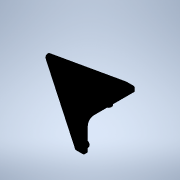
# Autodesk Inventor part: gato
Saved by Autodesk Inventor 2021 (Build 250183000, 183)
## iProperties
Created: 2024-10-06
Part Number: gato
Material: Generic
Document SubType Name: Modeling
Designer: hojan
Density: 1 g/cm^3
Appearance: Default
Author: hojan
Autodesk Inventor part; units mm, degrees
ref_plane "YZ Plane" through (0, 0, 0) normal (1, 0, 0) x (0, 1, 0)
ref_plane "XZ Plane" through (0, 0, 0) normal (0, 1, 0) x (-1, 0, 0)
ref_plane "XY Plane" through (0, 0, 0) normal (0, 0, 1) x (1, 0, 0)
sketch "Boceto1" plane through (0, 0, 0) normal (1, 0, 0) x (0, 1, 0)
  circle A0 centre (0, 0) radius 2.5
  line L0 (2.5, 0) -> (2.5, 10.6639)
  line L1 (2.5, 2.5) -> (-7.5, 2.5)
  line L2 (-7.5, 2.5) -> (-9.5, 2.5)
  line L3 (-9.5, 2.5) -> (-9.5, 4.5)
  line L4 (-9.5, 4.5) -> (2.5, 4.5)
  line L5 (0, 0) -> (-4.5773, -4.5773)
  line L6 (0, 0) -> (6.4732, 0) construction
  circle A1 centre (0, 0) radius 2.5
  line L7 (0, 2.5) -> (10.6639, 2.5)
  line L8 (2.5, 2.5) -> (2.5, -7.5)
  line L9 (2.5, -7.5) -> (2.5, -9.5)
  line L10 (2.5, -9.5) -> (4.5, -9.5)
  line L11 (4.5, -9.5) -> (4.5, 2.5)
  line L12 (2.5, 4.5) -> (4.5, 4.5)
  line L13 (4.5, 4.5) -> (4.5, 2.5)
  point P0 (0, 2.5)
  dimension "d0" = 5
  dimension "d1" = 10
  dimension "d2" = 2
  dimension "d3" = 2
  dimension "d4" = 135
  constraints: 28 end point, 6 symmetric about line, 4 point on line, 3 horizontal, 3 perpendicular, 2 coincident, 2 vertical, 1 equal length, 1 vertical alignment, 6 other
  measures "d1" distance of L1.start L1.end
  measures "d2" distance of L1.end L2.end
  measures "d3" distance of L2.end L3.end
  measures "d4" angle of L5 L6
extrude "Extrusión1" add sketch "Boceto1" along normal blind 3 contours A0 L1 L0 | L0 L7 L11 L10 L9 L8 | L1 L2 L3 L4 L0 | L0 L12 L13 L7
sketch "Boceto2" plane through (3, 0, 0) normal (1, 0, 0) x (0, 0, -1)
  line L0 (16.7965, 4.5) -> (-17.9745, 33.0686)
  line L1 (-4.5, 4.5) -> (-4.5, -9.5) projected
  line L2 (-17.9745, 33.0686) -> (-4.5, -9.5)
  line L3 (-2.5, -9.5) -> (-2.5, 0) projected
  arc A0 (0, 2.5) -> (-2.5, 0) centre (0, 0) ccw projected
  line L4 (0, 2.5) -> (9.5, 2.5) projected
  line L5 (9.5, 2.5) -> (9.5, 4.5) projected
  line L6 (9.5, 4.5) -> (-4.5, 4.5) projected
  line L7 (-4.5, 4.5) -> (-4.5, -9.5) projected
  line L8 (-4.5, -9.5) -> (-2.5, -9.5) projected
  line L9 (9.5, 2.5) -> (9.5, 4.5) projected
  line L10 (9.5, 4.5) -> (16.7965, 4.5)
  line L11 (16.7965, 2.5) -> (9.5, 2.5)
  line L12 (9.5, 2.5) -> (16.7965, 2.5)
  line L13 (16.7965, 4.5) -> (16.7965, 2.5)
  constraints: 12 end point, 2 perpendicular, 1 collinear, 1 horizontal
extrude "Extrusión2" add sketch "Boceto2" against normal blind 3 contours L10 L6 L1 L2 L0 | L13 L11 L5 L10
sketch "Boceto3" plane through (0, 2.5, -9.5) normal (0, -1, 0) x (1, 0, 0)
  line L0 (0, 0) -> (3, 0) projected
  line L1 (1.5, 0) -> (1.5, 2)
  circle A0 centre (1.5, 2) radius 1.35
  point P0 (0, 9.5)
  dimension "d9" = 2
  dimension "d10" = 2.7
  constraints: 2 end point, 1 centre point, 1 coincident, 1 midpoint, 1 vertical
  measures "d9" distance of L1.start L1.end
  measures "d10" diameter of A0
extrude "Extrusión3" add sketch "Boceto3" along normal blind 1
fillet "Empalme1" radius 0.2 1 edges at (0.15, 1.5, -7.5)
sketch "Boceto4" plane through (0, -9.5, 2.5) normal (0, 0, -1) x (-1, 0, 0)
  line L0 (0, 0) -> (-3, 0) projected
  line L1 (-1.5, 0) -> (-1.5, 2)
  circle A0 centre (-1.5, 2) radius 1.35
  point P0 (0, 9.5)
  dimension "d14" = 2
  dimension "d15" = 2.7
  constraints: 2 end point, 1 centre point, 1 coincident, 1 midpoint, 1 vertical
  measures "d14" distance of L1.start L1.end
  measures "d15" diameter of A0
extrude "Extrusión4" add sketch "Boceto4" along normal blind 1
fillet "Empalme2" radius 0.2 1 edges at (2.85, -7.5, 1.5)
fillet "Empalme3" radius 1 3 edges at (1.5, 4.5, -16.7965) (1.5, -9.5, 4.5) (1.5, 33.0686, 17.9745)
